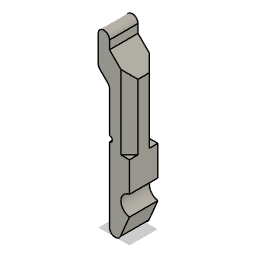
_penhouder lever.3cee7135-46d6-436c-b803-6f9b700ddbff (Autodesk Fusion 360 design; units mm, degrees)
Autodesk Fusion 360 part; units mm, degrees
sketch "Sketch1" plane through (0, 0, 0) normal (0, 0, 1) x (1, 0, 0)
  circle A0 centre (0, 0) radius 3.5
  line L0 (-11.5, 49) -> (-11.5, 37)
  line L1 (-0.5, -3.4641) -> (-0.5, 37)
  line L2 (-0.5, -3.4641) -> (-7.5, -20)
  circle A1 centre (-7.5, 16.9115) radius 1
  line L3 (-11.5, 49) -> (-7.5, 49)
  line L4 (-11.5, 37) -> (-7.5, 33)
  line L5 (-7.5, 44) -> (-0.5, 37)
  line L6 (-7.5, -20) -> (-7.5, 33)
  line L7 (-7.5, 44) -> (-7.5, 49)
  point P0 (-7.5, 16.9115)
  dimension "d1" = 7
  dimension "d2" = 4
  dimension "d6" = 0.5
  dimension "d7" = 20
  dimension "d8" = 7
  dimension "d9" = 18.5
  dimension "d10" = 2
  dimension "d11" = 69
  dimension "d12" = 12
  dimension "d14" = 5
  dimension "d26" = 45
  constraint coincident A0.centre origin
  constraint vertical L6
  constraint parallel L0 L6
  constraint vertical L1
  constraint coincident A0 L1.start
  constraint coincident P0 L6
  constraint coincident P0 A1.centre
  constraint coincident L5.start L6
  constraint collinear L6 L7
  constraint perpendicular L0 L3
  constraint parallel L4 L5
  measures "d1" diameter of A0
  measures "d2" distance of L0 L6
  measures "d6" distance of A0.centre L1
  measures "d7" vertical distance of A0.centre L2.end
  measures "d8" distance of L1 L6
  measures "d9" distance of A0.centre P0
  measures "d10" diameter of A1
  measures "d11" vertical distance of L2.end L0.start
  measures "d12" distance of L0.start L0.end
  measures "d14" distance of L3.end L5.start
  measures "d26" angle of L5 L6
extrude "Extrude1" add sketch "Sketch1" along normal blind 10 contours A0 L0 L1 L2 A1 L3 L4 L5 L6 L7
sketch "Sketch2" plane through (0, 49, 0) normal (0, 1, 0) x (-1, 0, 0)
  line L0 (7.5, 0) -> (11.5, 0)
  line L1 (11.5, 0) -> (11.5, 10)
  line L2 (11.5, 10) -> (7.5, 10)
  line L3 (7.5, 10) -> (7.5, 0)
  line L4 (3.5, 0) -> (-1.5, 5)
  line L5 (-1.5, 5) -> (3.5, 10)
  line L6 (7.5, 0) -> (0.5, 0)
  line L7 (3.5, 10) -> (-2, 10)
  line L8 (-2, 10) -> (-2, 0)
  line L9 (-2, 0) -> (3.5, 0)
  line L10 (0.5, 10) -> (7.5, 10)
  point P0 (0.5, 0)
  point P1 (0.5, 10)
  dimension "d17" = 3
  dimension "d18" = 3
  dimension "d19" = 45
  constraint perpendicular L4 L5
  constraint coincident L4.start L6
  constraint horizontal L7
  constraint perpendicular L7 L8
  constraint perpendicular L8 L9
  constraint coincident L5.end L10
  measures "d17" distance of L4.start P0
  measures "d18" horizontal distance of L5.end P1
  measures "d19" angle of L4 L6
extrude "Extrude2" cut sketch "Sketch2" against normal blind 35 contours L4 L5 L6 L7 L8 L9 L10
fillet "Fillet1" radius 2 2 edges at (-11.5, 49, 5) (-7.5, 49, 5)
fillet "Fillet2" radius 2 3 edges at (-7.5, 33, 5) (-11.5, 37, 5) (-7.5, -20, 5)
